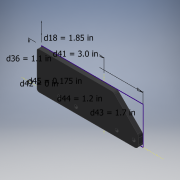
# Autodesk Inventor part: J005548
Saved by Autodesk Inventor 2018.2 (Build 222227000, 227)
## iProperties
Created: 2015-12-16
Material: ACRYLIC, BLACK
Vendor: HHMI: JRC - ID&F
Document SubType Name: Modeling
Designer: ARNOLDJ
Density: 1 g/cm^3
Appearance: Generic
Description: NRB TREADMILL SIDE WALL
Project: COMMON
Part Number: J005548
RuleStatus: InUse
AfterDocSave0: file://Part Number Cleaner
LAB/DEPT: COMMON
REQUESTING SCIENTIST: COMMON
SURFACE ROUGHNESS: N/A
DESIGN DEPARTMENT: HHMI: JRC - ID&F
SPECIAL FINISH: NONE
ALTERED ITEM PART NUMBER: N/A
ALTERED ITEM VENDOR: N/A
ALTERED ITEM DESCRIPTION: N/A
Author: ARNOLDJ
Revision Number: A
Autodesk Inventor part; units mm, degrees
ref_plane "YZ Plane" through (0, 0, 0) normal (1, 0, 0) x (0, 1, 0)
ref_plane "XZ Plane" through (0, 0, 0) normal (0, 1, 0) x (-1, 0, 0)
ref_plane "XY Plane" through (0, 0, 0) normal (0, 0, 1) x (1, 0, 0)
sketch "Sketch1" plane through (0, 0, 0) normal (0, 0, 1) x (1, 0, 0)
  line L0 (0, 33.528) -> (0, -5.588) construction
  line L1 (-62.23, 0) -> (44.45, 0) construction
  line L2 (29.21, 0) -> (-46.99, 0)
  line L3 (-46.99, 0) -> (-46.99, 27.94)
  line L4 (-46.99, 27.94) -> (29.21, 27.94)
  line L5 (29.21, 0) -> (29.21, 27.94)
  point P0 (0, 0)
  point P1 (12.7, 4.445)
  point P2 (-30.48, 4.445)
  dimension "d18" = 46.99
  dimension "d36" = 27.94
  dimension "d41" = 76.2
  dimension "d42" = 0
  dimension "d43" = 43.18
  dimension "d44" = 30.48
  dimension "d45" = 4.445
  constraints: 8 end point, 2 perpendicular, 2 point on line, 1 vertical
  measures "d18" distance between parallel lines of L0 L3
  measures "d36" distance of L2.end L3.end
  measures "d41" distance of L3.end L4.end
  measures "d42" distance between parallel lines of L1 L2
  measures "d43" distance of point (12.7, 4.445) point (-30.48, 4.445)
  measures "d44" distance from line of point (-30.48, 4.445) L0
  measures "d45" distance from line of point (-30.48, 4.445) L1
extrude "Extrusion1" add sketch "Sketch1" along normal blind 3.175
hole "Hole1" at (-30.48, 4.445, 0) at (12.7, 4.445, 0) direction (0, 0, 1) diameter 2.4638 depth 8.7884 tip angle 118
fillet "Fillet1" radius 1.5875 2 edges at (-46.99, 27.94, 1.5875) (-46.99, 0, 1.5875)
chamfer "Chamfer1" distance 19.05 angle 45 1 edges at (29.21, 27.94, 1.5875)
fillet "Fillet2" radius 3.175 3 edges at (10.16, 27.94, 1.5875) (29.21, 0, 1.5875) (29.21, 8.89, 1.5875)
pattern_linear "Rectangular Pattern1" count 2 spacing 12.7 along (1, 0, 0) of "Hole1"
body "Solid1"
